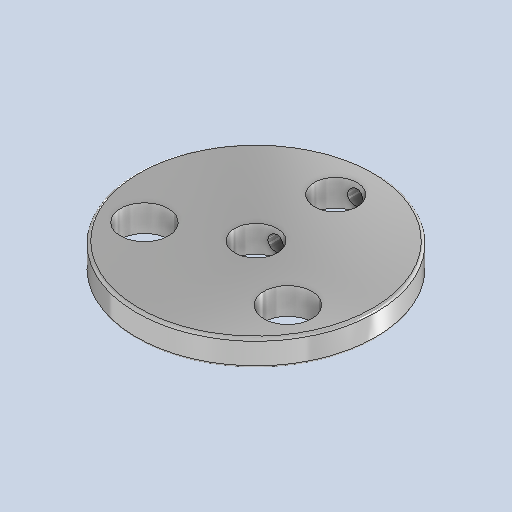
# Autodesk Inventor part: 201 part 3
Saved by Autodesk Inventor 2025.1 (Build 291241000, 241)
## iProperties
Created: 2024-08-01
Part Number: 201 part 3
Material: Aluminum 6061-AHC
Document SubType Name: Modeling
Designer: ffogue
Density: 2.7 g/cm^3
Appearance: Aluminum - Dark
Author: ffogue
Autodesk Inventor part; units mm, degrees
ref_plane "YZ Plane" through (0, 0, 0) normal (1, 0, 0) x (0, 1, 0)
ref_plane "XY Plane" through (0, 0, 0) normal (0, 0, 1) x (1, 0, 0)
sketch "Sketch1" plane through (0, 0, 0) normal (0, 0, 1) x (1, 0, 0)
  circle A0 centre (0, 0) radius 22.5
  dimension "d0" = 45
  constraints: 1 centre point, 1 coincident
  measures "d0" diameter of A0
extrude "Extrusion1" add sketch "Sketch1" along normal mid plane 5
sketch "Sketch2" plane through (0, 0, 2.5) normal (0, 0, 1) x (1, 0, 0)
  circle A0 centre (0, 0) radius 4
  circle A1 centre (0, 15) radius 4
  circle A2 centre (-13.5, -7.5) radius 4.5
  circle A3 centre (13.5, -7.5) radius 4.5
  dimension "d3" = 8
  dimension "d4" = 15
  dimension "d5" = 8
  dimension "d6" = 7.5
  dimension "d7" = 13.5
  dimension "d8" = 13.5
  dimension "d9" = 9
  dimension "d10" = 9
  constraints: 4 centre point, 1 coincident, 1 horizontal alignment, 1 vertical alignment
  measures "d3" diameter of A0
  measures "d4" distance of point (0, 0) A1.centre
  measures "d5" diameter of A1
  measures "d6" vertical distance of A3.centre point (0, 0)
  measures "d7" horizontal distance of point (0, 0) A3.centre
  measures "d8" horizontal distance of point (0, 0) A2.centre
  measures "d9" diameter of A2
  measures "d10" diameter of A3
extrude "Extrusion2" cut sketch "Sketch2" against normal up to surface (5 mm away)
fillet "Fillet1" radius 0.5 2 edges at (-22.5, 0, 2.5) (-22.5, 0, -2.5)
ref_plane "Work Plane1" through (0, 3, 0) normal (0, 1, 0) x (-1, 0, 0)
sketch "Sketch3" plane through (0, 3, 0) normal (0, 1, 0) x (-1, 0, 0)
  line L0 (-4, 2.5) -> (4, 2.5) projected
  line L1 (4, -2.5) -> (-4, -2.5) projected
  line L2 (22.5, 2) -> (-22.5, 2) projected
  line L3 (-22.5, -2) -> (22.5, -2) projected
  line L4 (-22.5, -2) -> (-22.5, 2) projected
  line L5 (22.5, -2) -> (22.5, 2) projected
  point P0 (0, 0)
  point P1 (0, 0)
  point P2 (-22.5, 0)
  point P3 (0, -2)
  constraints: 2 midpoint, 1 coincident, 1 horizontal alignment, 1 vertical alignment
hole "Hole1" at (0, 3, 0) direction (0, 1, 0) diameter 3 end through all
equation "\"d8\" = d7"
equation "\"d10\" = d9"
equation "\"d11\" = d10"
body "Solid1"
